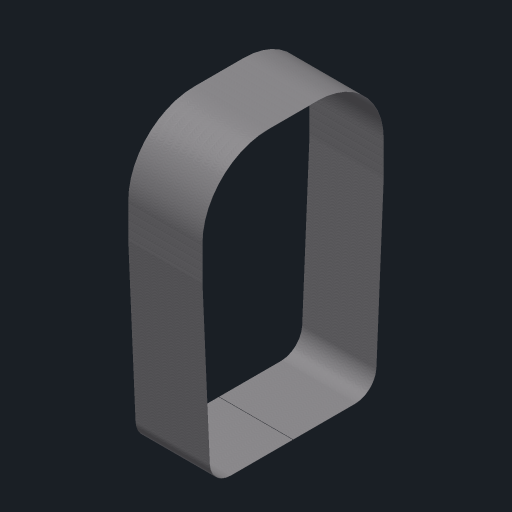
# Autodesk Inventor part: CARCASA_ALUM_1
Saved by Autodesk Inventor 2024.3 (Build 283343000, 343)
## iProperties
Created: 2024-05-14
Part Number: CARCASA_ALUM_1
Material: Steel, Mild, Welded
Document SubType Name: Sheet Metal
Designer: Niler
Density: 7.85 g/cm^3
Sheet Metal Rule: Default_mm
Appearance: Weld - Steel Mild
Flat Pattern Width: 45 cm
Flat Pattern Length: 507.527 cm
Flat Pattern Area: 22838.7 cm^2
Sheet Metal Width: 450.000 mm
Sheet Metal Length: 5075.266 mm
Sheet Metal Area: 2283869.554 mm^2
Author: Niler
Autodesk Inventor part; units mm, degrees
ref_plane "YZ Plane" through (0, 0, 0) normal (1, 0, 0) x (0, 1, 0)
ref_plane "XZ Plane" through (0, 0, 0) normal (0, 1, 0) x (-1, 0, 0)
ref_plane "XY Plane" through (0, 0, 0) normal (0, 0, 1) x (1, 0, 0)
sketch "Sketch1" plane through (0, 0, 0) normal (0, 1, 0) x (-1, 0, 0)
  line L0 (-225, 150) -> (225, 150)
  line L1 (225, 150) -> (225, -150)
  line L2 (225, -150) -> (-225, -150)
  line L3 (-225, -150) -> (-225, 150)
  line L4 (-225, 150) -> (225, -150) construction
  line L5 (225, 150) -> (-225, -150) construction
  point P0 (0, 0)
  dimension "d0" = 300
  dimension "d1" = 450
extrude "Plate1" add sketch "Sketch1" along normal blind 1.5
sketch "Sketch2" plane through (-225, -400, 550) normal (0, 0, 1) x (1, 0, 0)
  line L0 (450, 0) -> (0, 0)
  line L1 (0, 0) -> (0, -208.5)
  line L2 (0, -208.5) -> (450, -208.5)
  line L3 (450, -208.5) -> (450, 0)
  constraints: 6 end point, 1 horizontal, 1 perpendicular, 1 vertical
edge flange "Flange1" height 610 angle 90 thickness 1.5 bend radius 400 thickness toward (0, 0, 1) relief straight relief width 1.5 relief depth 0.75 corner gap 1.5 corner form 0 edges at (0, 0, 150) (0, 0, -150) wall of the first edge with corners at (225, -400, 550) (-225, -400, 550) (-225, -608.5, 550) (225, -608.5, 550)
bend "Bend1"
corner "Corner1"
sketch "Sketch3" plane through (-225, -608.5907, 549.9979) normal (0, -0.045363, 0.9989706) x (1, 0, 0)
  line L0 (450, 0) -> (0, 0)
  line L1 (0, 0) -> (0, -976.8646)
  line L2 (0, -976.8646) -> (450, -976.8646)
  line L3 (450, -976.8646) -> (450, 0)
  constraints: 6 end point, 1 horizontal, 1 perpendicular, 1 vertical
edge flange "Flange2" height 976.91 angle 2.6 thickness 1.5 bend radius 2 thickness toward (0, -0.045363, 0.9989706) relief straight relief width 1.5 relief depth 0.75 corner gap 1.5 corner form 0 edges at (0, -608.5, 550) (0, -608.5, -550) wall of the first edge with corners at (225, -608.5907, 549.9979) (-225, -608.5907, 549.9979) (-225, -1584.4497, 505.6844) (225, -1584.4497, 505.6844)
bend "Bend2"
corner "Corner2"
sketch "Sketch4" plane through (-225, -1707.1206, 377.3167) normal (0, -1, 0) x (1, 0, 0)
  line L0 (450, 0) -> (0, 0)
  line L1 (0, 0) -> (0, -375.7693)
  line L2 (0, -375.7693) -> (450, -375.7693)
  line L3 (450, -375.7693) -> (450, 0)
  constraints: 6 end point, 1 horizontal, 1 perpendicular, 1 vertical
edge flange "Flange3" height 500 angle 87.4 thickness 1.5 bend radius 128.5 thickness toward (0, -1, 0) relief straight relief width 1.5 relief depth 0.75 corner gap 1.5 corner form 0 edges at (0, -1584.4497, 505.6844) (0, -1584.4497, -505.6844) wall of the first edge with corners at (225, -1707.1206, 377.3167) (-225, -1707.1206, 377.3167) (-225, -1707.1206, 1.5474) (225, -1707.1206, 1.5474)
bend "Bend3"
corner "Corner3"
equation "\"d2\" = Thickness"
equation "\"d3\" = BendReliefWidth"
equation "\"d4\" = BendReliefDepth"
equation "\"d5\" = MinimumRemnant"
equation "\"d6\" = TransitionRadius"
equation "\"d10\" = CornerReliefSize"
equation "\"d11\" = GapSize"
equation "\"d12\" = JacobiRadiusSize"
equation "\"d13\" = BendReliefWidth"
equation "\"d14\" = BendReliefDepth"
equation "\"d15\" = MinimumRemnant"
equation "\"d16\" = TransitionRadius"
equation "\"d20\" = CornerReliefSize"
equation "\"d21\" = GapSize"
equation "\"d22\" = JacobiRadiusSize"
equation "\"d23\" = BendReliefWidth"
equation "\"d24\" = BendReliefDepth"
equation "\"d25\" = MinimumRemnant"
equation "\"d26\" = TransitionRadius"
equation "\"d30\" = CornerReliefSize"
equation "\"d31\" = GapSize"
equation "\"d32\" = JacobiRadiusSize"
equation "\"GapSize\" = Thickness"
equation "\"BendRadius\" = Thickness"
equation "\"MinimumRemnant\" = 2 * Thickness"
equation "\"BendReliefDepth\" = 0.5 * Thickness"
equation "\"BendReliefWidth\" = Thickness"
equation "\"CornerReliefSize\" = 4 * Thickness"
equation "\"JacobiRadiusSize\" = BendRadius"
equation "\"TransitionRadius\" = BendRadius"
equation "\"Thickness\" = 1.5"
body "Solid1"
